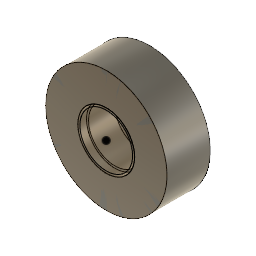
Drive Axis v2 (Autodesk Fusion 360 archive; units mm, degrees)
design "Hermosairis Crawler Tire Only 120mm"
Autodesk Fusion 360 part; units mm, degrees
note: some values were not read from the file. Chosen so that the rebuilt part matches the saved one: which face or edge a step refers to; how an offset face is resized. Set by a fixed rule: which sketch regions a step uses.
sketch "Sketch1" plane through (0, 0, 0) normal (0, 1, 0) x (1, 0, 0)
  circle A0 centre (0, 0) radius 60
  dimension "d1" = 120
  measures "d1" diameter of A0
extrude "Extrude1" add sketch "Sketch1" along normal blind 43
sketch "Sketch2" plane through (0, 0, 0) normal (0, -1, 0) x (1, 0, 0)
  circle A0 centre (0, 0) radius 60
  circle A1 centre (0, 0) radius 26
  circle A2 centre (0, 0) radius 28
  dimension "d4" = 52
  dimension "d7" = 2
  measures "d4" diameter of A1
extrude "Extrude3" cut sketch "Sketch2" against normal blind 8.5 contours A2
extrude "Extrude2" cut sketch "Sketch2" against normal up to surface (43 mm away) contours A1
sketch "Sketch3" plane through (0, 43, 0) normal (0, 1, 0) x (-1, 0, 0)
  circle A0 centre (0, 0) radius 26
  circle A1 centre (0, 0) radius 60
  circle A2 centre (0, 0) radius 28
  dimension "d10" = 2
extrude "Extrude4" cut sketch "Sketch3" against normal blind 8.5 contours A2

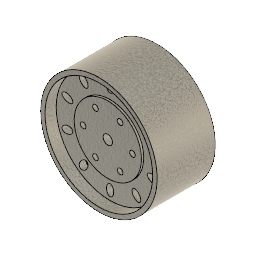
design "Hermosairis Crawler Rim 120mm"
Autodesk Fusion 360 part; units mm, degrees
sketch "Skizze1" plane through (0, 0, 0) normal (0, 1, 0) x (1, 0, 0)
  circle A0 centre (0, 0) radius 26
  dimension "d1" = 52
  measures "d1" diameter of A0
extrude "Extrusion1" add sketch "Skizze1" along normal blind 26 makes body 1
sketch "Skizze2" plane through (0, 0, 0) normal (0, -1, 0) x (1, 0, 0)
  circle A0 centre (0, 0) radius 26
  circle A1 centre (0, 0) radius 24
  dimension "d4" = 2
extrude "Extrude2" cut sketch "Skizze2" against normal blind 5 contours A1 bodies 1
sketch "Sketch3" plane through (0, 5, 0) normal (0, -1, 0) x (1, 0, 0)
  circle A0 centre (0, 0) radius 24
  circle A1 centre (0, 0) radius 15
extrude "Extrude3" add sketch "Sketch3" along normal blind 1 contours A1 bodies 1
sketch "Sketch4" plane through (0, 4, 0) normal (0, -1, 0) x (1, 0, 0)
  circle A0 centre (0, 0) radius 15
  circle A1 centre (0, 0) radius 2.1
  dimension "d9" = 4.2
  measures "d9" diameter of A1
extrude "Extrude4" cut sketch "Sketch4" against normal up to surface (22 mm away) contours A1 bodies 1
sketch "Sketch5" plane through (0, 4, 0) normal (0, -1, 0) x (1, 0, 0)
  circle A0 centre (0, 0) radius 2.1
  circle A1 centre (0, 0) radius 15
  circle A2 centre (0, 0) radius 11 construction
  circle A3 centre (-11, 0) radius 1.25
  circle A4 centre (-5.5, -9.5263) radius 1.25
  circle A5 centre (5.5, -9.5263) radius 1.25
  circle A6 centre (11, 0) radius 1.25
  circle A7 centre (5.5, 9.5263) radius 1.25
  circle A8 centre (-5.5, 9.5263) radius 1.25
  dimension "d12" = 2.5
  dimension "d14" = 360
  measures "d12" diameter of A3
extrude "Extrude5" cut sketch "Sketch5" against normal up to surface (22 mm away) contours A3 | A4 | A5 | A6 | A7 | A8 bodies 1
sketch "Sketch6" plane through (0, 5, 0) normal (0, -1, 0) x (1, 0, 0)
  circle A0 centre (0, 0) radius 15
  circle A1 centre (0, 0) radius 24
  circle A2 centre (0, 0) radius 20 construction
  ellipse E0 centre (0, 20) end of major axis (0, 17.5) minor radius 1.6029
  line L0 (0, 22.5) -> (0, 17.5)
  line L1 (-1.6029, 20) -> (1.6029, 20)
  ellipse E1 centre (-11.7557, 16.1803) end of major axis (-10.2862, 14.1578) minor radius 1.6029
  ellipse E2 centre (-19.0211, 6.1803) end of major axis (-16.6435, 5.4078) minor radius 1.6029
  ellipse E3 centre (-19.0211, -6.1803) end of major axis (-16.6435, -5.4078) minor radius 1.6029
  ellipse E4 centre (-11.7557, -16.1803) end of major axis (-10.2862, -14.1578) minor radius 1.6029
  ellipse E5 centre (0, -20) end of major axis (0, -17.5) minor radius 1.6029
  ellipse E6 centre (11.7557, -16.1803) end of major axis (10.2862, -14.1578) minor radius 1.6029
  ellipse E7 centre (19.0211, -6.1803) end of major axis (16.6435, -5.4078) minor radius 1.6029
  ellipse E8 centre (19.0211, 6.1803) end of major axis (16.6435, 5.4078) minor radius 1.6029
  ellipse E9 centre (11.7557, 16.1803) end of major axis (10.2862, 14.1578) minor radius 1.6029
  dimension "d17" = 40
  dimension "d19" = 360
  measures "d17" diameter of A2
extrude "Extrude6" cut sketch "Sketch6" against normal blind 3 contours E0 L0 L1 | E0 L0 L1 | E0 L0 L1 | E0 L0 L1 | E1 | E2 | E3 | E4 | E5 | E6 | E7 | E8 | E9 bodies 1
sketch "Sketch7" plane through (0, 26, 0) normal (0, 1, 0) x (-1, 0, 0)
  circle A0 centre (-5.5, -9.5263) radius 1.25
  circle A1 centre (5.5, 9.5263) radius 1.25
  circle A2 centre (5.5, -9.5263) radius 1.25
  circle A3 centre (-11, 0) radius 1.25
  circle A4 centre (-5.5, 9.5263) radius 1.25
  circle A5 centre (11, 0) radius 1.25
  circle A6 centre (0, 0) radius 2.1
  circle A7 centre (0, 0) radius 26
  circle A8 centre (0, 0) radius 23.5
  dimension "d23" = 2.5
extrude "Extrude7" cut sketch "Sketch7" against normal blind 10 contours A8 bodies 1
sketch "Sketch8" plane through (0, 16, 0) normal (0, 1, 0) x (-1, 0, 0)
  circle A0 centre (0, 0) radius 2.1
  circle A1 centre (11, 0) radius 1.25
  circle A2 centre (-5.5, 9.5263) radius 1.25
  circle A3 centre (-11, 0) radius 1.25
  circle A4 centre (5.5, -9.5263) radius 1.25
  circle A5 centre (5.5, 9.5263) radius 1.25
  circle A6 centre (-5.5, -9.5263) radius 1.25
  circle A7 centre (0, 0) radius 23.5
  line L0 (-6, 0) -> (-3, -5.1962)
  line L1 (-3, -5.1962) -> (3, -5.1962)
  line L2 (3, -5.1962) -> (6, 0)
  line L3 (6, 0) -> (3, 5.1962)
  line L4 (3, 5.1962) -> (-3, 5.1962)
  line L5 (-3, 5.1962) -> (-6, 0)
  dimension "d27" = 6
  measures "d27" distance of A0.centre
extrude "Extrude8" cut sketch "Sketch8" against normal blind 5 contours L0 L1 L2 L3 L4 L5 bodies 1
copy_body "Body->Comp1" bodies 1 removing the originals makes body 2 in component "Rim"
component "Rim" placed x (1, 0, 0) y (0, 1, 0) z (0, 0, 1) at (0, 0, 0)

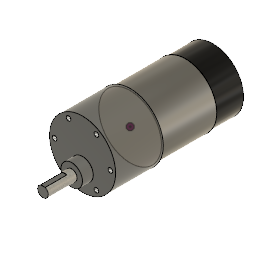
design "37D 131-1 Gearbox Motor"
Autodesk Fusion 360 part; units mm, degrees
sketch "Skizze1" plane through (0, 0, 0) normal (0, 1, 0) x (1, 0, 0)
  circle A0 centre (0, 0) radius 17.4
  dimension "d1" = 34.8
  dimension "d62" = 0
  dimension "d63" = 0
  dimension "d64" = 0
  dimension "d65" = 0
  dimension "d74" = 0
  dimension "d75" = 0
  dimension "d76" = 0
  dimension "d77" = 0
  dimension "d86" = 0
  dimension "d87" = 0
  dimension "d88" = 0
  dimension "d89" = 0
  measures "d1" diameter of A0
extrude "Extrusion3" add sketch "Skizze1" along normal blind 30.7 makes body 1
extrude "Extrusion2" add sketch "Skizze1" along normal blind 30.7 separate body makes body 2
extrude "Extrusion1" add sketch "Skizze1" along normal blind 30.7 separate body makes body 3
copy_body "Körper->Berechn1" bodies 1 removing the originals makes body 4 in component "Motor"
ref_plane "Arbeitsebene1" through (0, 0, 0) normal (0, 1, 0) x (1, 0, 0) in component "Gearbox"
sketch "Skizze1 (2)" plane through (0, 0, 0) normal (0, 1, 0) x (1, 0, 0) in component "Gearbox"
  circle A0 centre (0, 0) radius 18.4
  dimension "d13" = 36.8
  measures "d13" diameter of A0
extrude "Extrusion1'" add sketch "Skizze1 (2)" against normal blind 26.5 separate body makes body 5 in component "Gearbox"
ref_plane "Arbeitsebene1" through (0, 30.7, 0) normal (0, 1, 0) x (1, 0, 0) in component "Encoder"
sketch "Skizze1 (3)" plane through (0, 30.7, 0) normal (0, 1, 0) x (1, 0, 0) in component "Encoder"
  circle A0 centre (0, 0) radius 17
  dimension "d17" = 34
  measures "d17" diameter of A0
extrude "Extrusion1''" add sketch "Skizze1 (3)" along normal blind 15.4 separate body makes body 6 in component "Encoder"
sketch "Skizze3" plane through (0, -26.5, 0) normal (0, -1, 0) x (1, 0, 0)
  circle A0 centre (0, 0) radius 18.4
  circle A1 centre (0, 0) radius 15.5 construction
  circle A2 centre (0, -7) radius 6
  line L0 (0, 0) -> (0, -28) construction
  dimension "d20" = 31
  dimension "d21" = 12
  dimension "d22" = 7
  measures "d20" diameter of A1
  measures "d21" diameter of A2
  measures "d22" distance of A0.centre
extrude "Extrusion2'" add sketch "Skizze3" along normal blind 6 contours A2 bodies 5 in component "Gearbox"
sketch "Skizze4" plane through (0, -32.5, 0) normal (0, -1, 0) x (1, 0, 0)
  circle A0 centre (0, -7) radius 6
  circle A1 centre (0, -7) radius 3
  dimension "d25" = 6
  measures "d25" diameter of A1
extrude "Extrusion3'" add sketch "Skizze4" along normal blind 16 contours A1 bodies 5 in component "Gearbox"
sketch "Skizze2" plane through (0, -26.5, 0) normal (0, -1, 0) x (1, 0, 0) in component "Gearbox"
  circle A0 centre (0, -7) radius 6
  circle A1 centre (0, 0) radius 18.4
  circle A2 centre (0, 0) radius 15.5 construction
  circle A3 centre (-15.5, 0) radius 1.6
  circle A4 centre (-7.75, -13.4234) radius 1.6
  circle A5 centre (7.75, -13.4234) radius 1.6
  circle A6 centre (15.5, 0) radius 1.6
  circle A7 centre (7.75, 13.4234) radius 1.6
  circle A8 centre (-7.75, 13.4234) radius 1.6
  dimension "d28" = 31
  dimension "d29" = 3.2
  dimension "d31" = 360
  measures "d28" diameter of A2
  measures "d29" diameter of A3
extrude "Extrusion4" cut sketch "Skizze2" against normal blind 3 contours A3 | A4 | A5 | A6 | A7 | A8 bodies 5 in component "Gearbox"
thread "Gewinde1" "ISO Metric profile 3.0 M3x0.5 6H" major diameter 3.086 minor diameter 2.529 pitch 0.5 angle 60 resizes the face on face at (-6.152, -24.5, 13.3436) on bodies 5 in component "Gearbox"
thread "Gewinde2" "ISO Metric profile 3.0 M3x0.5 6H" major diameter 3.086 minor diameter 2.529 pitch 0.5 angle 60 resizes the face on face at (9.348, -24.5, 13.3436) on bodies 5 in component "Gearbox"
thread "Gewinde3" "ISO Metric profile 3.0 M3x0.5 6H" major diameter 3.086 minor diameter 2.529 pitch 0.5 angle 60 resizes the face on face at (17.098, -24.5, -0.0798) on bodies 5 in component "Gearbox"
thread "Gewinde4" "ISO Metric profile 3.0 M3x0.5 6H" major diameter 3.086 minor diameter 2.529 pitch 0.5 angle 60 resizes the face on face at (-13.902, -24.5, -0.0798) on bodies 5 in component "Gearbox"
thread "Gewinde5" "ISO Metric profile 3.0 M3x0.5 6H" major diameter 3.086 minor diameter 2.529 pitch 0.5 angle 60 resizes the face on face at (-6.152, -24.5, -13.5031) on bodies 5 in component "Gearbox"
thread "Gewinde6" "ISO Metric profile 3.0 M3x0.5 6H" major diameter 3.086 minor diameter 2.529 pitch 0.5 angle 60 resizes the face on face at (9.348, -24.5, -13.5031) on bodies 5 in component "Gearbox"
sketch "Skizze5" plane through (0, -48.5, 0) normal (0, -1, 0) x (1, 0, 0)
  circle A0 centre (0, -7) radius 3
  line L0 (-3, -2.3) -> (3, -2.3)
  line L1 (3, -2.3) -> (3, -4.3)
  line L2 (3, -4.3) -> (-3, -4.3)
  line L3 (-3, -4.3) -> (-3, -2.3)
  dimension "d130" = 2.7
extrude "Extrusion5" cut sketch "Skizze5" against normal blind 12 contours A0 L2 | A0 L0 L1 L2 L3 picked at (-0.0644, -4.105) bodies 5 in component "Gearbox"
component "Motor" placed x (1, 0, 0) y (0, 1, 0) z (0, 0, 1) at (0, 0, 0)
component "Gearbox" placed x (1, 0, 0) y (0, 1, 0) z (0, 0, 1) at (0, 0, 0)
component "Encoder" placed x (1, 0, 0) y (0, 1, 0) z (0, 0, 1) at (0, 0, 0)
